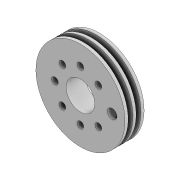
# Autodesk Inventor part: Motor_pulley
Saved by Autodesk Inventor 2022 (Build 260153000, 153)
## iProperties
Created: 2022-07-09
Part Number: Motor_pulley
Material: Generic
Document SubType Name: Modeling
Designer: dell
Density: 1 g/cm^3
Appearance: Default
Author: dell
Autodesk Inventor part; units mm, degrees
ref_plane "YZ Plane" through (0, 0, 0) normal (1, 0, 0) x (0, 1, 0)
ref_plane "XZ Plane" through (0, 0, 0) normal (0, 1, 0) x (-1, 0, 0)
ref_plane "XY Plane" through (0, 0, 0) normal (0, 0, 1) x (1, 0, 0)
sketch "Sketch1" plane through (0, 0, 0) normal (1, 0, 0) x (0, 1, 0)
  line L0 (0, 3) -> (14, 3)
  line L1 (14, 3) -> (14, -0.5)
  line L2 (14, -0.5) -> (0, -0.5)
  line L3 (0, -0.5) -> (0, 3)
  line L4 (0, -1.7) -> (0, 6.7) projected
  line L5 (14, 2) -> (14, 0.5)
  line L6 (14, 0.5) -> (10, 0.5)
  line L7 (10, 0.5) -> (10, 2)
  line L8 (10, 2) -> (14, 2)
  line L9 (10, 3) -> (10, 4.5)
  line L10 (10, 4.5) -> (14, 4.5)
  line L11 (14, 4.5) -> (14, 5.5)
  line L12 (14, 5.5) -> (0, 5.5)
  point P0 (0, 0)
  dimension "d0" = 3.5
  dimension "d1" = 3
  dimension "d2" = 14
  dimension "d4" = 1
  dimension "d5" = 1
  dimension "d19" = 4
  dimension "d26" = 1.5
  dimension "d27" = 1
  constraints: 24 end point, 6 parallel, 5 point on line, 2 collinear, 2 horizontal, 2 perpendicular, 2 vertical
  measures "d0" distance of L2.end L0.start
  measures "d1" distance from line of point (0, 0) L0
  measures "d2" distance between parallel lines of L1 L3
  measures "d4" distance from line of L0 L5.start
  measures "d5" distance of L1.end L5.end
  measures "d19" distance of L5.end L6.end
  measures "d26" distance of L9.start L9.end
  measures "d27" distance between parallel lines of L10 L12
revolve "Revolution1" add sketch "Sketch1" angle 360 about axis through (0, 0, -10) along (0, 0, 1) contours L4 L12 L11 L10 L9 L0 | L0 L1 L8 L7 L6 L2 L3
sketch "Sketch2" plane through (0, 0, -0.5) normal (0, 0, -1) x (-1, 0, 0)
  circle A0 centre (0, 8) radius 1.05
  circle A1 centre (0, 0) radius 4.5
  dimension "d7" = 2.1
  dimension "d8" = 8
  dimension "d9" = 9
  constraints: 2 centre point, 1 coincident
  measures "d7" diameter of A0
  measures "d8" distance of point (0, 0) A0.centre
  measures "d9" diameter of A1
extrude "Extrusion1" cut sketch "Sketch2" against normal blind 100
pattern_circular "Circular Pattern1" count 8 over 360 about axis through (0, 0, -10) along (0, 0, 1) of "Extrusion1"
sketch "Sketch3" plane through (0, 0, -0.5) normal (0, 0, -1) x (-1, 0, 0)
  circle A0 centre (-10, 0) radius 1.5
  circle A1 centre (-8, 0) radius 1.05 projected
  point P0 (0, 0)
  point P1 (-8.7131, -0.7707)
  point P2 (-8.7131, 0.7707)
  dimension "d15" = 3
  dimension "d16" = 10
  constraints: 1 centre point
  measures "d15" diameter of A0
  measures "d16" distance of point (0, 0) A0.centre
extrude "Extrusion2" add sketch "Sketch3" against normal blind 6
extrude "Extrusion5" cut sketch "Sketch3" against normal blind 100 contours A0 A1 | A1 A0 picked at (-8.689, 0.1306) picked at (-10.6732, 0.0411)
body "Solid1"
